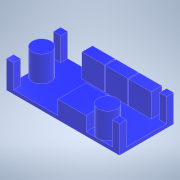
# Autodesk Inventor part: LM2596 Buck Converter
Saved by Autodesk Inventor 2022 (Build 260153000, 153)
## iProperties
Created: 2021-09-22
Part Number: LM2596 Buck Converter
Material: Generic
Document SubType Name: Modeling
Designer: tecware
Density: 1 g/cm^3
Appearance: Smooth - Navy
Author: tecware
Autodesk Inventor part; units mm, degrees
ref_plane "YZ Plane" through (0, 0, 0) normal (1, 0, 0) x (0, 1, 0)
ref_plane "XZ Plane" through (0, 0, 0) normal (0, 1, 0) x (-1, 0, 0)
ref_plane "XY Plane" through (0, 0, 0) normal (0, 0, 1) x (1, 0, 0)
sketch "Sketch1" plane through (0, 0, 0) normal (0, 1, 0) x (-1, 0, 0)
  line L0 (0, -23.07) -> (-48.1, -23.07)
  line L1 (-48.1, -23.07) -> (-48.1, 0)
  line L2 (-48.1, 0) -> (0, 0)
  line L3 (0, 0) -> (0, -23.07)
  point P0 (0, 0)
  dimension "d0" = 48.1
  dimension "d1" = 23.07
  constraints: 8 end point, 2 parallel, 1 horizontal, 1 perpendicular
  measures "d0" distance of L1.end L2.end
  measures "d1" distance of L0.end L1.end
extrude "Extrusion1" add sketch "Sketch1" along normal blind 1.6
sketch "Sketch2" plane through (0, 1.6, 0) normal (0, 1, 0) x (1, 0, 0)
  line L0 (33.6, 23.07) -> (43.1, 23.07)
  line L1 (43.1, 23.07) -> (43.1, 18.57)
  line L2 (43.1, 18.57) -> (33.6, 18.57)
  line L3 (33.6, 18.57) -> (33.6, 23.07)
  line L4 (48.1, 23.07) -> (0, 23.07) projected
  line L5 (48.1, 0) -> (48.1, 23.07) projected
  line L6 (23.6, 23.07) -> (33.1, 23.07)
  line L7 (33.1, 23.07) -> (33.1, 18.57)
  line L8 (33.1, 18.57) -> (23.6, 18.57)
  line L9 (23.6, 18.57) -> (23.6, 23.07)
  line L10 (13.6, 23.07) -> (23.1, 23.07)
  line L11 (23.1, 23.07) -> (23.1, 18.57)
  line L12 (23.1, 18.57) -> (13.6, 18.57)
  line L13 (13.6, 18.57) -> (13.6, 23.07)
  point P0 (0, 0)
  dimension "d4" = 9.5
  dimension "d5" = 4.5
  dimension "d6" = 5
  dimension "d7" = 9.5
  dimension "d8" = 4.5
  dimension "d9" = 0.5
  dimension "d10" = 9.5
  dimension "d11" = 4.5
  dimension "d12" = 0.5
  constraints: 24 end point, 6 parallel, 3 collinear, 3 horizontal, 3 perpendicular
  measures "d4" distance of L1.end L2.end
  measures "d5" distance of L0.end L1.end
  measures "d6" distance between parallel lines of L5 L1
  measures "d7" distance of L7.end L8.end
  measures "d8" distance of L6.end L7.end
  measures "d9" distance between parallel lines of L3 L7
  measures "d10" distance of L11.end L12.end
  measures "d11" distance of L10.end L11.end
  measures "d12" distance between parallel lines of L9 L11
extrude "Extrusion2" add sketch "Sketch2" along normal blind 10
sketch "Sketch3" plane through (0, 1.6, 0) normal (0, 1, 0) x (1, 0, 0)
  line L0 (48.1, 0) -> (48.1, 23.07) projected
  line L1 (48.1, 23.07) -> (45.1, 23.07)
  line L2 (45.1, 23.07) -> (45.1, 20.07)
  line L3 (45.1, 20.07) -> (48.1, 20.07)
  line L4 (48.1, 20.07) -> (48.1, 23.07)
  line L5 (0, 23.07) -> (3, 23.07)
  line L6 (3, 23.07) -> (3, 20.07)
  line L7 (3, 20.07) -> (0, 20.07)
  line L8 (0, 20.07) -> (0, 23.07)
  line L9 (0, 0) -> (3, 0)
  line L10 (3, 0) -> (3, 3)
  line L11 (3, 3) -> (0, 3)
  line L12 (0, 3) -> (0, 0)
  line L13 (48.1, 0) -> (45.1, 0)
  line L14 (45.1, 0) -> (45.1, 3)
  line L15 (45.1, 3) -> (48.1, 3)
  line L16 (48.1, 3) -> (48.1, 0)
  dimension "d15" = 3
  dimension "d16" = 3
  dimension "d17" = 3
  constraints: 32 end point, 8 parallel, 4 horizontal, 4 perpendicular, 3 point on line
  measures "d15" distance of L3.end L2.end
  measures "d16" distance of L2.end L1.end
  measures "d17" distance of L5.end L6.end
extrude "Extrusion3" add sketch "Sketch3" along normal blind 10
sketch "Sketch4" plane through (0, 1.6, 0) normal (0, 1, 0) x (1, 0, 0)
  circle A0 centre (39.1, 4) radius 4
  line L0 (48.1, 3) -> (48.1, 20.07) projected
  circle A1 centre (4, 11) radius 4
  point P0 (0, 0)
  dimension "d20" = 8
  dimension "d21" = 9
  dimension "d22" = 8
  constraints: 2 centre point
  measures "d20" diameter of A0
  measures "d21" distance from line of L0 A0.centre
  measures "d22" diameter of A1
extrude "Extrusion4" add sketch "Sketch4" along normal blind 11
sketch "Sketch5" plane through (0, 1.6, 0) normal (0, 1, 0) x (1, 0, 0)
  line L0 (21.9, 12.1) -> (33.9, 12.1)
  line L1 (33.9, 12.1) -> (33.9, 0)
  line L2 (33.9, 0) -> (21.9, 0)
  line L3 (21.9, 0) -> (21.9, 12.1)
  circle A0 centre (39.1, 4) radius 4 projected
  point P0 (0, 0)
  dimension "d25" = 12
  dimension "d26" = 12.1
  dimension "d27" = 1.2
  constraints: 8 end point, 2 parallel, 1 horizontal, 1 perpendicular
  measures "d25" distance of L1.end L2.end
  measures "d26" distance of L0.end L1.end
  measures "d27" distance edge to line of A0 L1
extrude "Extrusion5" add sketch "Sketch5" along normal blind 6 contours L0 L1 L2 L3
body "Solid1"
